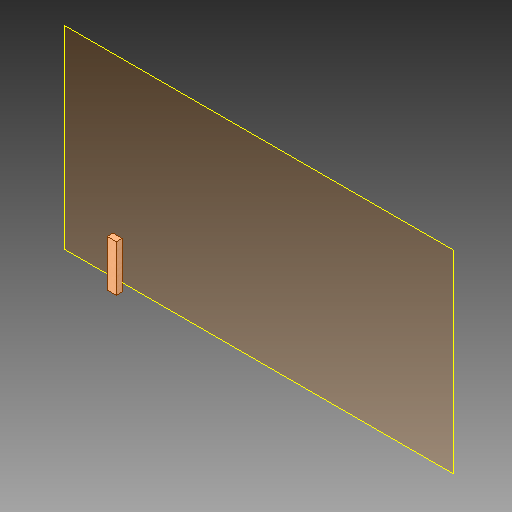
# Autodesk Inventor part: beam
Saved by Autodesk Inventor 2019.3 (Build 233278000, 278)
## iProperties
Created: 2020-09-24
Part Number: beam
Material: Holz (Kirsche)
Document SubType Name: Modeling
Designer: Nicolas Frick
Density: 0.63 g/cm^3
Appearance: Kirsche - natur - schwacher Glanz
Author: Nicolas Frick
Autodesk Inventor part; units mm, degrees
ref_plane "YZ Plane" through (0, 0, 0) normal (1, 0, 0) x (0, 1, 0)
ref_plane "XZ Plane" through (0, 0, 0) normal (0, 1, 0) x (-1, 0, 0)
ref_plane "XY Plane" through (0, 0, 0) normal (0, 0, 1) x (1, 0, 0)
ref_plane "Arbeitsebene1" through (0, 0, 0) normal (0, 0, 1) x (1, 0, 0)
sketch "Skizze1" plane through (0, 0, 0) normal (0, 0, 1) x (1, 0, 0)
  line L0 (901.5, 442.5) -> (901.5, -442.5) construction
  line L1 (901.5, -442.5) -> (-901.5, -442.5) construction
  line L2 (-901.5, -442.5) -> (-901.5, 442.5) construction
  line L3 (-901.5, 442.5) -> (901.5, 442.5) construction
  line L4 (914, 455) -> (-914, 455) construction
  line L5 (-914, 455) -> (-914, -455) construction
  line L6 (-914, -455) -> (914, -455) construction
  line L7 (914, -455) -> (914, 455) construction
  line L8 (-734.2086, -542.5) -> (-717.297, -542.5) construction
  line L9 (-706.1667, -542.5) -> (-754.1364, -542.5)
  line L10 (-754.1364, -542.5) -> (-754.1364, -302.9215)
  line L11 (-754.1364, -302.9215) -> (-706.1667, -302.9215)
  line L12 (-706.1667, -302.9215) -> (-706.1667, -542.5)
  point P0 (0, 0)
  constraints: 8 end point, 2 parallel, 1 horizontal, 1 perpendicular
extrude "Extrusion1" add sketch "Skizze1" along normal blind 30
